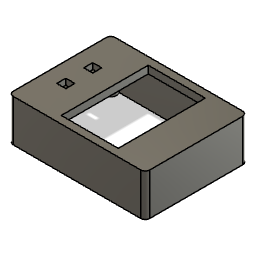
Enclosure_V2 (Autodesk Fusion 360 design; units mm, degrees)
Autodesk Fusion 360 part; units mm, degrees
sketch "Sketch1" plane through (0, 0, 0) normal (0, 1, 0) x (1, 0, 0) in component "Base"
  line L0 (88, -34) -> (-88, -34)
  line L1 (-88, -34) -> (-88, 34)
  line L2 (-88, 34) -> (88, 34)
  line L3 (88, 34) -> (88, -34)
  line L4 (88, -34) -> (-88, 34) construction
  line L5 (-88, -34) -> (88, 34) construction
  line L6 (85.5, -31.5) -> (-85.5, -31.5)
  line L7 (-85.5, -31.5) -> (-85.5, 31.5)
  line L8 (-85.5, 31.5) -> (85.5, 31.5)
  line L9 (85.5, 31.5) -> (85.5, -31.5)
  dimension "d2" = 176
  dimension "d3" = 68
  dimension "d4" = 2.5
  constraint perpendicular L0 L1
  constraint parallel L0 L2
  constraint parallel L1 L3
  constraint horizontal L0
  constraint coincident L4 origin
  constraint coincident L5 origin
  measures "d2" distance of L1.end L2.end
  measures "d3" distance of L0.end L1.end
extrude "Extrude1" add sketch "Sketch1" along normal blind 23 contours L0 L1 L2 L3 | L6 L7 L8 L9 makes body 1 in component "Base"
sketch "Sketch2" plane through (0, 23, 0) normal (0, 1, 0) x (-1, 0, 0) in component "Base"
  line L0 (-88, -34) -> (88, -34)
  line L1 (88, -34) -> (88, 34)
  line L2 (88, 34) -> (-88, 34)
  line L3 (-88, 34) -> (-88, -34)
  line L4 (85.5, 31.5) -> (-85.5, 31.5)
  line L5 (-85.5, 31.5) -> (-85.5, -31.5)
  line L6 (-85.5, -31.5) -> (85.5, -31.5)
  line L7 (85.5, -31.5) -> (85.5, 31.5)
  circle A0 centre (-83, -29) radius 2
  circle A1 centre (-83, 29) radius 2
  circle A2 centre (0, 29) radius 2
  circle A3 centre (0, -29) radius 2
  circle A4 centre (83, -29) radius 2
  circle A5 centre (83, 29) radius 2
  dimension "d7" = -2.5
  dimension "d62" = 4
  dimension "d63" = 5
  dimension "d64" = 5
  dimension "d65" = 4
  dimension "d66" = 5
  dimension "d67" = 5
  dimension "d68" = 4
  dimension "d69" = 5
  dimension "d70" = 4
  dimension "d71" = 5
  dimension "d72" = 4
  dimension "d73" = 5
  dimension "d74" = 5
  dimension "d75" = 4
  dimension "d76" = 5
  dimension "d77" = 5
  measures "d62" diameter of A0
  measures "d63" distance of L0 A0.centre
  measures "d64" distance of L3 A0.centre
  measures "d65" diameter of A1
  measures "d66" distance of L3 A1.centre
  measures "d67" distance of L2 A1.centre
  measures "d68" diameter of A2
  measures "d69" distance of L2 A2.centre
  measures "d70" diameter of A3
  measures "d71" distance of L0 A3.centre
  measures "d72" diameter of A4
  measures "d73" distance of L0 A4.centre
  measures "d74" distance of L1 A4.centre
  measures "d75" diameter of A5
  measures "d76" distance of L2 A5.centre
  measures "d77" distance of L1 A5.centre
extrude "Extrude2" cut sketch "Sketch2" against normal up to surface (19 mm away) contours L4 L5 L6 L7 | A0 | A1 | A2 | A3 | A4 | A5 bodies 1 in component "Base"
fillet "Fillet1" radius 2 4 edges at (85.5, 13.5, -31.5) (85.5, 13.5, 31.5) (-85.5, 13.5, 31.5) (-85.5, 13.5, -31.5) on bodies 1 in component "Base"
fillet "Fillet2" radius 3 4 edges at (-88, 11.5, 34) (-88, 11.5, -34) (88, 11.5, -34) (88, 11.5, 34) on bodies 1 in component "Base"
sketch "Sketch3" plane through (0, 0, 0) normal (0, -1, 0) x (1, 0, 0) in component "Base"
  arc A0 (88, 31) -> (85, 34) centre (85, 31) ccw
  line L0 (85, 34) -> (-85, 34)
  arc A1 (-85, 34) -> (-88, 31) centre (-85, 31) ccw
  line L1 (-88, 31) -> (-88, -31) construction
  arc A2 (-88, -31) -> (-85, -34) centre (-85, -31) ccw
  line L2 (-85, -34) -> (85, -34)
  arc A3 (85, -34) -> (88, -31) centre (85, -31) ccw
  line L3 (88, -31) -> (88, 31)
sketch "Sketch4" plane through (0, 0, 0) normal (0, -1, 0) x (1, 0, 0) in component "Base"
  arc A0 (88, 31) -> (85, 34) centre (85, 31) ccw
  line L0 (85, 34) -> (-85, 34)
  arc A1 (-85, 34) -> (-88, 31) centre (-85, 31) ccw
  line L1 (-88, 31) -> (-88, -31)
  arc A2 (-88, -31) -> (-85, -34) centre (-85, -31) ccw
  line L2 (-85, -34) -> (85, -34)
  arc A3 (85, -34) -> (88, -31) centre (85, -31) ccw
  line L3 (88, -31) -> (88, 31)
  circle A4 centre (-61.5, 24) radius 1.75
  line L4 (85, 34) -> (-85, 34)
  circle A5 centre (-61.5, -24.5) radius 1.75
  line L5 (-85, -34) -> (85, -34)
  circle A6 centre (-28.5, 24) radius 1.75
  circle A7 centre (-28.5, -24.5) radius 1.75
  circle A8 centre (-61.5, 24) radius 3.5
  circle A9 centre (-28.5, 24) radius 3.5
  circle A10 centre (-61.5, -24.5) radius 3.5
  circle A11 centre (-28.5, -24.5) radius 3.5
  circle A12 centre (-83, 29) radius 4
  circle A13 centre (-83, 29) radius 2
  circle A14 centre (-83, 29) radius 4
  circle A15 centre (-83, 29) radius 2.1
  circle A16 centre (-83, -29) radius 2
  line L6 (-88, 31) -> (-88, -31)
  circle A17 centre (-83, -29) radius 4
  circle A18 centre (0, 29) radius 4
  circle A19 centre (0, 29) radius 2
  circle A20 centre (0, -29) radius 4
  circle A21 centre (0, -29) radius 2
  circle A22 centre (83, 29) radius 4
  line L7 (88, -31) -> (88, 31)
  circle A23 centre (83, 29) radius 2
  circle A24 centre (83, -29) radius 4
  circle A25 centre (83, -29) radius 2
  dimension "d14" = 3.5
  dimension "d15" = 26.5
  dimension "d16" = 10
  dimension "d17" = 3.5
  dimension "d18" = 26.5
  dimension "d20" = 3.5
  dimension "d21" = 59.5
  dimension "d22" = 10
  dimension "d23" = 3.5
  dimension "d24" = 59.5
  dimension "d26" = 7
  dimension "d27" = 7
  dimension "d28" = 7
  dimension "d29" = 7
  dimension "d36" = 8
  dimension "d37" = 5
  dimension "d38" = 5
  dimension "d39" = 4
  dimension "d40" = 8
  dimension "d41" = 4.2
  dimension "d42" = 4
  dimension "d43" = 5
  dimension "d44" = 5
  dimension "d45" = 8
  dimension "d46" = 8
  dimension "d47" = 5
  dimension "d48" = 4
  dimension "d49" = 8
  dimension "d50" = 5
  dimension "d51" = 4
  dimension "d52" = 8
  dimension "d53" = 5
  dimension "d54" = 5
  dimension "d55" = 4
  dimension "d56" = 8
  dimension "d57" = 5
  dimension "d58" = 5
  dimension "d59" = 4
  dimension "d154" = 48.5
  dimension "d155" = 48.5
  constraint concentric A4 A8
  constraint concentric A6 A9
  constraint concentric A5 A10
  constraint concentric A7 A11
  constraint concentric A12 A13
  constraint concentric A14 A15
  constraint concentric A16 A17
  constraint concentric A18 A19
  constraint concentric A20 A21
  constraint concentric A22 A23
  constraint concentric A24 A25
  measures "d14" diameter of A4
  measures "d15" distance of L1 A4.centre
  measures "d16" distance of A4.centre L4
  measures "d17" diameter of A5
  measures "d18" distance of L1 A5.centre
  measures "d20" diameter of A6
  measures "d21" distance of L1 A6.centre
  measures "d22" distance of L4 A6.centre
  measures "d23" diameter of A7
  measures "d24" distance of L1 A7.centre
  measures "d26" diameter of A8
  measures "d27" diameter of A9
  measures "d28" diameter of A10
  measures "d29" diameter of A11
  measures "d36" diameter of A12
  measures "d37" distance of L4 A12.centre
  measures "d38" distance of L1 A12.centre
  measures "d39" diameter of A13
  measures "d40" diameter of A14
  measures "d41" diameter of A15
  measures "d42" diameter of A16
  measures "d43" distance of A16.centre L6
  measures "d44" distance of L5 A16.centre
  measures "d45" diameter of A17
  measures "d46" diameter of A18
  measures "d47" distance of L0 A18.centre
  measures "d48" diameter of A19
  measures "d49" diameter of A20
  measures "d50" distance of L5 A20.centre
  measures "d51" diameter of A21
  measures "d52" diameter of A22
  measures "d53" distance of A22.centre L7
  measures "d54" distance of L4 A22.centre
  measures "d55" diameter of A23
  measures "d56" diameter of A24
  measures "d57" distance of L3 A24.centre
  measures "d58" distance of L5 A24.centre
  measures "d59" diameter of A25
  measures "d154" distance of A6.centre A7.centre
  measures "d155" distance of A4.centre A5.centre
extrude "Extrude6" add sketch "Sketch4" against normal blind 23 contours A12 A14 | A13 | A15 | A16 | A17 | A18 | A19 | A20 | A21 | A22 | A23 | A24 | A25 bodies 1 in component "Base"
extrude "Extrude4" cut sketch "Sketch4" against normal up to surface (4 mm away) contours A4 | A5 | A6 | A7 bodies 1 in component "Base"
extrude "Extrude5" cut sketch "Sketch4" against normal blind 2.5 contours A8 | A9 | A10 | A11 bodies 1 in component "Base"
sketch "Sketch5" plane through (0, 0, 0) normal (0, -1, 0) x (1, 0, 0) in component "Base"
  circle A0 centre (-28.5, 24) radius 3.5
  circle A1 centre (-61.5, -24.5) radius 3.5
  circle A2 centre (-61.5, 24) radius 3.5
  circle A3 centre (-28.5, -24.5) radius 3.5
  arc A4 (88, 31) -> (85, 34) centre (85, 31) ccw
  line L0 (85, 34) -> (-85, 34)
  arc A5 (-85, 34) -> (-88, 31) centre (-85, 31) ccw
  line L1 (-88, 31) -> (-88, -31)
  arc A6 (-88, -31) -> (-85, -34) centre (-85, -31) ccw
  line L2 (-85, -34) -> (85, -34)
  arc A7 (85, -34) -> (88, -31) centre (85, -31) ccw
  line L3 (88, -31) -> (88, 31)
  line L4 (-2, 25) -> (2, 25)
  line L5 (2, 25) -> (2, -25)
  line L6 (2, -25) -> (-2, -25)
  line L7 (-2, -25) -> (-2, 25)
  constraint horizontal L4
  constraint vertical L5
  constraint horizontal L6
  constraint vertical L7
sketch "Sketch2 (2)" plane through (0, 23, 0) normal (0, 1, 0) x (-1, 0, 0) in component "Lid1"
  arc A0 (-85, 34) -> (-88, 31) centre (-85, 31) ccw
  line L0 (-88, 31) -> (-88, -31)
  arc A1 (-88, -31) -> (-85, -34) centre (-85, -31) ccw
  line L1 (-85, -34) -> (85, -34)
  arc A2 (85, -34) -> (88, -31) centre (85, -31) ccw
  line L2 (88, -31) -> (88, 31)
  arc A3 (88, 31) -> (85, 34) centre (85, 31) ccw
  line L3 (85, 34) -> (-85, 34)
  arc A4 (-85.5, 25.8775) -> (-79.8775, 31.5) centre (-83, 29) ccw
  line L4 (-79.8775, 31.5) -> (-3.1225, 31.5)
  arc A5 (-3.1225, 31.5) -> (3.1225, 31.5) centre (0, 29) ccw
  line L5 (3.1225, 31.5) -> (79.8775, 31.5)
  arc A6 (79.8775, 31.5) -> (85.5, 25.8775) centre (83, 29) ccw
  line L6 (85.5, 25.8775) -> (85.5, -25.8775)
  arc A7 (85.5, -25.8775) -> (79.8775, -31.5) centre (83, -29) ccw
  line L7 (79.8775, -31.5) -> (3.1225, -31.5)
  arc A8 (3.1225, -31.5) -> (-3.1225, -31.5) centre (0, -29) ccw
  line L8 (-3.1225, -31.5) -> (-79.8775, -31.5)
  arc A9 (-79.8775, -31.5) -> (-85.5, -25.8775) centre (-83, -29) ccw
  line L9 (-85.5, -25.8775) -> (-85.5, 25.8775)
  line L10 (85, -34) -> (-85, -34)
  arc A10 (85, -34) -> (88, -31) centre (85, -31) ccw
  line L11 (88, 31) -> (88, -31)
  arc A11 (88, 31) -> (85, 34) centre (85, 31) ccw
  line L12 (-85, 34) -> (85, 34)
  line L13 (-88, -31) -> (-88, 31)
  arc A12 (-85, 34) -> (-88, 31) centre (-85, 31) ccw
  arc A13 (-88, -31) -> (-85, -34) centre (-85, -31) ccw
  point P0 (85, -34)
  point P1 (88, -31)
  point P2 (88, 31)
  point P3 (85, 34)
  point P4 (-85, 34)
  point P5 (-88, 31)
  point P6 (-88, -31)
  point P7 (-85, -34)
extrude "Extrude2'" add sketch "Sketch2 (2)" along normal blind 6 separate body contours A0 L0 A1 L1 A2 L2 A3 L3 L10 A10 L11 A11 L12 L13 A12 A13 | A4 L4 A5 L5 A6 L6 A7 L7 A8 L8 A9 L9 makes body 2 in component "Lid1"
sketch "Sketch5 (2)" plane through (0, 23, 0) normal (0, 1, 0) x (-1, 0, 0) in component "Lid1"
  arc A0 (-85, 34) -> (-88, 31) centre (-85, 31) ccw
  line L0 (-88, 31) -> (-88, -31)
  arc A1 (-88, -31) -> (-85, -34) centre (-85, -31) ccw
  line L1 (-85, -34) -> (85, -34)
  arc A2 (85, -34) -> (88, -31) centre (85, -31) ccw
  line L2 (88, -31) -> (88, 31)
  arc A3 (88, 31) -> (85, 34) centre (85, 31) ccw
  line L3 (85, 34) -> (-85, 34)
  arc A4 (-85.5, 25.8775) -> (-79.8775, 31.5) centre (-83, 29) ccw
  line L4 (-79.8775, 31.5) -> (-3.1225, 31.5)
  arc A5 (-3.1225, 31.5) -> (3.1225, 31.5) centre (0, 29) ccw
  line L5 (3.1225, 31.5) -> (79.8775, 31.5)
  arc A6 (79.8775, 31.5) -> (85.5, 25.8775) centre (83, 29) ccw
  line L6 (85.5, 25.8775) -> (85.5, -25.8775)
  arc A7 (85.5, -25.8775) -> (79.8775, -31.5) centre (83, -29) ccw
  line L7 (79.8775, -31.5) -> (3.1225, -31.5)
  arc A8 (3.1225, -31.5) -> (-3.1225, -31.5) centre (0, -29) ccw
  line L8 (-3.1225, -31.5) -> (-79.8775, -31.5)
  arc A9 (-79.8775, -31.5) -> (-85.5, -25.8775) centre (-83, -29) ccw
  line L9 (-85.5, -25.8775) -> (-85.5, 25.8775)
  arc A10 (85.5, -25.8775) -> (79.8775, -31.5) centre (83, -29) ccw
  line L10 (79.8775, -31.5) -> (3.1225, -31.5)
  arc A11 (3.1225, -31.5) -> (-3.1225, -31.5) centre (0, -29) ccw
  line L11 (-3.1225, -31.5) -> (-79.8775, -31.5)
  arc A12 (-79.8775, -31.5) -> (-85.5, -25.8775) centre (-83, -29) ccw
  line L12 (-85.5, -25.8775) -> (-85.5, 25.8775)
  arc A13 (-85.5, 25.8775) -> (-79.8775, 31.5) centre (-83, 29) ccw
  line L13 (-79.8775, 31.5) -> (-3.1225, 31.5)
  arc A14 (-3.1225, 31.5) -> (3.1225, 31.5) centre (0, 29) ccw
  line L14 (3.1225, 31.5) -> (79.8775, 31.5)
  arc A15 (79.8775, 31.5) -> (85.5, 25.8775) centre (83, 29) ccw
  line L15 (85.5, 25.8775) -> (85.5, -25.8775)
  point P0 (79.8775, -31.5)
  point P1 (3.1225, -31.5)
  point P2 (-3.1225, -31.5)
  point P3 (-79.8775, -31.5)
  point P4 (-85.5, -25.8775)
  point P5 (-85.5, 25.8775)
  point P6 (-79.8775, 31.5)
  point P7 (-3.1225, 31.5)
  point P8 (3.1225, 31.5)
  point P9 (79.8775, 31.5)
  point P10 (85.5, -25.8775)
  point P11 (85.5, 25.8775)
sketch "Sketch6" plane through (0, 23, 0) normal (0, 1, 0) x (-1, 0, 0) in component "Lid1"
  arc A0 (-85, 34) -> (-88, 31) centre (-85, 31) ccw
  line L0 (-88, 31) -> (-88, -31)
  arc A1 (-88, -31) -> (-85, -34) centre (-85, -31) ccw
  line L1 (-85, -34) -> (85, -34)
  arc A2 (85, -34) -> (88, -31) centre (85, -31) ccw
  line L2 (88, -31) -> (88, 31)
  arc A3 (88, 31) -> (85, 34) centre (85, 31) ccw
  line L3 (85, 34) -> (-85, 34)
  arc A4 (-85.5, 25.8775) -> (-79.8775, 31.5) centre (-83, 29) ccw
  line L4 (-79.8775, 31.5) -> (-3.1225, 31.5)
  arc A5 (-3.1225, 31.5) -> (3.1225, 31.5) centre (0, 29) ccw
  line L5 (3.1225, 31.5) -> (79.8775, 31.5)
  arc A6 (79.8775, 31.5) -> (85.5, 25.8775) centre (83, 29) ccw
  line L6 (85.5, 25.8775) -> (85.5, -25.8775)
  arc A7 (85.5, -25.8775) -> (79.8775, -31.5) centre (83, -29) ccw
  line L7 (79.8775, -31.5) -> (3.1225, -31.5)
  arc A8 (3.1225, -31.5) -> (-3.1225, -31.5) centre (0, -29) ccw
  line L8 (-3.1225, -31.5) -> (-79.8775, -31.5)
  arc A9 (-79.8775, -31.5) -> (-85.5, -25.8775) centre (-83, -29) ccw
  line L9 (-85.5, -25.8775) -> (-85.5, 25.8775)
  line L10 (0, 25) -> (0, -25)
  constraint midpoint A5 L10.start
  constraint midpoint A8 L10.end
extrude "Extrude5'" cut sketch "Sketch6" along normal up to surface (6 mm away) contours A5 L5 A6 L6 A7 L7 A8 L10 bodies 2 in component "Lid1"
extrude "Extrude7" cut sketch "Sketch2" against normal blind 3 contours A0 | A1 | A2 | A3 | A4 | A5 bodies 1 in component "Base"
sketch "Sketch10" plane through (0, 0, 0) normal (0, -1, 0) x (1, 0, 0) in component "Base"
  circle A0 centre (-28.5, 24) radius 3.5
  circle A1 centre (-61.5, -24.5) radius 3.5
  circle A2 centre (-61.5, 24) radius 3.5
  circle A3 centre (-28.5, -24.5) radius 3.5
  arc A4 (88, 31) -> (85, 34) centre (85, 31) ccw
  line L0 (85, 34) -> (-85, 34)
  arc A5 (-85, 34) -> (-88, 31) centre (-85, 31) ccw
  line L1 (-88, 31) -> (-88, -31)
  arc A6 (-88, -31) -> (-85, -34) centre (-85, -31) ccw
  line L2 (-85, -34) -> (85, -34)
  arc A7 (85, -34) -> (88, -31) centre (85, -31) ccw
  line L3 (88, -31) -> (88, 31)
  line L4 (10, 19) -> (25, 19)
  line L5 (25, 19) -> (25, 4)
  line L6 (25, 4) -> (10, 4)
  line L7 (10, 4) -> (10, 19)
  line L8 (88, -31) -> (88, 31)
  line L9 (85, 34) -> (-85, 34)
  dimension "d137" = 15
  dimension "d138" = 15
  dimension "d140" = 78
  dimension "d143" = 15
  constraint horizontal L4
  constraint vertical L5
  constraint horizontal L6
  constraint vertical L7
  measures "d137" distance of L4.start L4.end
  measures "d138" distance of L4.start L6.end
  measures "d140" distance of L7 L8
  measures "d143" distance of L4 L9
extrude "Extrude12" cut sketch "Sketch10" against normal up to surface (4 mm away) contours L4 L5 L6 L7 bodies 1 in component "Base"
sketch "Sketch7" plane through (0, 23, 0) normal (0, 1, 0) x (-1, 0, 0) in component "Lid1"
  circle A0 centre (0, 29) radius 2
  circle A1 centre (83, -29) radius 2
  circle A2 centre (-83, -29) radius 2
  circle A3 centre (0, -29) radius 2
  circle A4 centre (83, 29) radius 2
  circle A5 centre (-83, 29) radius 2
  arc A6 (-85, 34) -> (-88, 31) centre (-85, 31) ccw
  line L0 (-88, 31) -> (-88, -31)
  arc A7 (-88, -31) -> (-85, -34) centre (-85, -31) ccw
  line L1 (-85, -34) -> (85, -34)
  arc A8 (85, -34) -> (88, -31) centre (85, -31) ccw
  line L2 (88, -31) -> (88, 31)
  arc A9 (88, 31) -> (85, 34) centre (85, 31) ccw
  line L3 (85, 34) -> (-85, 34)
  arc A10 (-85.5, 25.8775) -> (-79.8775, 31.5) centre (-83, 29) ccw
  line L4 (-79.8775, 31.5) -> (-3.1225, 31.5)
  arc A11 (-3.1225, 31.5) -> (3.1225, 31.5) centre (0, 29) ccw
  line L5 (3.1225, 31.5) -> (79.8775, 31.5)
  arc A12 (79.8775, 31.5) -> (85.5, 25.8775) centre (83, 29) ccw
  line L6 (85.5, 25.8775) -> (85.5, -25.8775)
  arc A13 (85.5, -25.8775) -> (79.8775, -31.5) centre (83, -29) ccw
  line L7 (79.8775, -31.5) -> (3.1225, -31.5)
  arc A14 (3.1225, -31.5) -> (-3.1225, -31.5) centre (0, -29) ccw
  line L8 (-3.1225, -31.5) -> (-79.8775, -31.5)
  arc A15 (-79.8775, -31.5) -> (-85.5, -25.8775) centre (-83, -29) ccw
  line L9 (-85.5, -25.8775) -> (-85.5, 25.8775)
  circle A16 centre (0, 29) radius 2
  circle A17 centre (-83, 29) radius 2
  circle A18 centre (-83, -29) radius 2
  circle A19 centre (0, -29) radius 2
  circle A20 centre (83, -29) radius 2
  circle A21 centre (83, 29) radius 2
  dimension "d92" = 4
  dimension "d93" = 4
  dimension "d94" = 4
  dimension "d95" = 4
  dimension "d96" = 4
  dimension "d97" = 4
  constraint concentric A0 A16
  constraint concentric A5 A17
  constraint concentric A2 A18
  constraint concentric A3 A19
  constraint concentric A1 A20
  constraint concentric A4 A21
  measures "d92" diameter of A16
  measures "d93" diameter of A17
  measures "d94" diameter of A18
  measures "d95" diameter of A19
  measures "d96" diameter of A20
  measures "d97" diameter of A21
extrude "Extrude4'" cut sketch "Sketch7" along normal blind 3 contours A0 A16 | A1 A20 | A2 A18 | A3 A19 | A4 A21 | A5 A17 bodies 2 in component "Lid1"
sketch "Sketch6 (2)" plane through (0, 0, 0) normal (0, -1, 0) x (1, 0, 0) in component "Base"
  circle A0 centre (-28.5, -24.5) radius 3.5
  circle A1 centre (-61.5, 24) radius 3.5
  circle A2 centre (-61.5, -24.5) radius 3.5
  circle A3 centre (-28.5, 24) radius 3.5
  line L0 (-2, 27) -> (2, 27)
  line L1 (2, 27) -> (2, -27)
  line L2 (2, -27) -> (-2, -27)
  line L3 (-2, -27) -> (-2, 27)
  line L4 (10, 4) -> (10, 19)
  line L5 (10, 19) -> (25, 19)
  line L6 (25, 19) -> (25, 4)
  line L7 (25, 4) -> (10, 4)
  arc A4 (88, 31) -> (85, 34) centre (85, 31) ccw
  line L8 (85, 34) -> (-85, 34)
  arc A5 (-85, 34) -> (-88, 31) centre (-85, 31) ccw
  line L9 (-88, 31) -> (-88, -31)
  arc A6 (-88, -31) -> (-85, -34) centre (-85, -31) ccw
  line L10 (-85, -34) -> (85, -34)
  arc A7 (85, -34) -> (88, -31) centre (85, -31) ccw
  line L11 (88, -31) -> (88, 31)
  constraint horizontal L0
  constraint vertical L1
  constraint horizontal L2
  constraint vertical L3
extrude "Extrude9" add sketch "Sketch6 (2)" against normal blind 23 contours L0 L1 L2 L3 bodies 1 in component "Base"
sketch "Sketch7 (2)" plane through (0, 23, 0) normal (0, 1, 0) x (-1, 0, 0) in component "Base"
  arc A0 (2, 25.5359) -> (3.1225, 31.5) centre (0, 29) ccw
  line L0 (3.1225, 31.5) -> (79.8775, 31.5)
  arc A1 (79.8775, 31.5) -> (85.5, 25.8775) centre (83, 29) ccw
  line L1 (85.5, 25.8775) -> (85.5, -25.8775)
  arc A2 (85.5, -25.8775) -> (79.8775, -31.5) centre (83, -29) ccw
  line L2 (79.8775, -31.5) -> (3.1225, -31.5)
  arc A3 (3.1225, -31.5) -> (2, -25.5359) centre (0, -29) ccw
  line L3 (2, -25.5359) -> (2, 25.5359)
  line L4 (-2, 25.5359) -> (-2, -25.5359)
  arc A4 (-2, -25.5359) -> (-3.1225, -31.5) centre (0, -29) ccw
  line L5 (-3.1225, -31.5) -> (-79.8775, -31.5)
  arc A5 (-79.8775, -31.5) -> (-85.5, -25.8775) centre (-83, -29) ccw
  line L6 (-85.5, -25.8775) -> (-85.5, 25.8775)
  arc A6 (-85.5, 25.8775) -> (-79.8775, 31.5) centre (-83, 29) ccw
  line L7 (-79.8775, 31.5) -> (-3.1225, 31.5)
  arc A7 (-3.1225, 31.5) -> (-2, 25.5359) centre (0, 29) ccw
  circle A8 centre (0, -29) radius 2
  circle A9 centre (0, 29) radius 2
  circle A10 centre (83, -29) radius 2
  circle A11 centre (-83, -29) radius 2
  circle A12 centre (83, 29) radius 2
  circle A13 centre (-83, 29) radius 2
  arc A14 (-85, 34) -> (-88, 31) centre (-85, 31) ccw
  line L8 (-88, 31) -> (-88, -31)
  arc A15 (-88, -31) -> (-85, -34) centre (-85, -31) ccw
  line L9 (-85, -34) -> (85, -34)
  arc A16 (85, -34) -> (88, -31) centre (85, -31) ccw
  line L10 (88, -31) -> (88, 31)
  arc A17 (88, 31) -> (85, 34) centre (85, 31) ccw
  line L11 (85, 34) -> (-85, 34)
  line L12 (2, -17) -> (-2, -17)
  line L13 (-2, -17) -> (-2, -14)
  line L14 (-2, -14) -> (2, -14)
  line L15 (2, -14) -> (2, -17)
  dimension "d120" = 17
  dimension "d121" = 3
  constraint horizontal L12
  constraint vertical L13
  constraint horizontal L14
  constraint vertical L15
  constraint coincident L4 L13.end
  constraint coincident L3 L12.start
  measures "d120" distance of L9 L12
  measures "d121" distance of L12 L14
extrude "Extrude10" cut sketch "Sketch7 (2)" against normal up to surface (19 mm away) contours L3 L4 L12 L13 L14 L15 bodies 1 in component "Base"
sketch "Sketch8" plane through (0, 0, 0) normal (0, -1, 0) x (1, 0, 0) in component "Base"
  circle A0 centre (-28.5, -24.5) radius 3.5
  circle A1 centre (-61.5, 24) radius 3.5
  circle A2 centre (-61.5, -24.5) radius 3.5
  circle A3 centre (-28.5, 24) radius 3.5
  line L0 (8, 27) -> (78, 27)
  line L1 (78, 27) -> (78, 24)
  line L2 (78, 24) -> (8, 24)
  line L3 (8, 24) -> (8, 27)
  line L4 (8, -27) -> (78, -27)
  line L5 (78, -27) -> (78, -24)
  line L6 (78, -24) -> (8, -24)
  line L7 (8, -24) -> (8, -27)
  line L8 (85, 34) -> (-85, 34)
  line L9 (88, -31) -> (88, 31)
  line L10 (-85, -34) -> (85, -34)
  line L11 (78, 27) -> (81, 27)
  line L12 (81, 27) -> (81, -27)
  line L13 (81, -27) -> (78, -27)
  line L14 (78, -27) -> (78, 27)
  line L15 (10, 4) -> (10, 19)
  line L16 (10, 19) -> (25, 19)
  line L17 (25, 19) -> (25, 4)
  line L18 (25, 4) -> (10, 4)
  arc A4 (88, 31) -> (85, 34) centre (85, 31) ccw
  line L19 (85, 34) -> (-85, 34)
  arc A5 (-85, 34) -> (-88, 31) centre (-85, 31) ccw
  line L20 (-88, 31) -> (-88, -31)
  arc A6 (-88, -31) -> (-85, -34) centre (-85, -31) ccw
  line L21 (-85, -34) -> (85, -34)
  arc A7 (85, -34) -> (88, -31) centre (85, -31) ccw
  line L22 (88, -31) -> (88, 31)
  dimension "d122" = 10
  dimension "d123" = 3
  dimension "d124" = 10
  dimension "d125" = 80
  dimension "d126" = 10
  dimension "d127" = 3
  dimension "d128" = 10
  dimension "d129" = 80
  dimension "d130" = 3
  constraint horizontal L0
  constraint vertical L1
  constraint horizontal L2
  constraint vertical L3
  constraint horizontal L4
  constraint vertical L5
  constraint horizontal L6
  constraint vertical L7
  constraint horizontal L11
  constraint vertical L12
  constraint horizontal L13
  constraint vertical L14
  measures "d122" distance of L2 L8
  measures "d123" distance of L0 L2
  measures "d124" distance of L1 L9
  measures "d125" distance of L3 L9
  measures "d126" distance of L6 L10
  measures "d127" distance of L4 L6
  measures "d128" distance of L5 L9
  measures "d129" distance of L7 L9
  measures "d130" distance of L0.end L11.end
extrude "Extrude11" add sketch "Sketch8" against normal blind 10 contours L0 L1 L2 L3 L14 | L1 L5 L11 L12 L13 L14 | L4 L5 L6 L7 L14 bodies 1 in component "Base"
sketch "Sketch1 (2)" plane through (0, 29, 0) normal (0, 1, 0) x (-1, 0, 0) in component "Lid2"
  line L0 (79.8775, -31.5) -> (3.1225, -31.5)
  arc A0 (3.1225, -31.5) -> (0, -25) centre (0, -29) ccw
  line L1 (0, -25) -> (0, 25)
  arc A1 (0, 25) -> (3.1225, 31.5) centre (0, 29) ccw
  line L2 (3.1225, 31.5) -> (79.8775, 31.5)
  arc A2 (79.8775, 31.5) -> (85.5, 25.8775) centre (83, 29) ccw
  line L3 (85.5, 25.8775) -> (85.5, -25.8775)
  arc A3 (85.5, -25.8775) -> (79.8775, -31.5) centre (83, -29) ccw
  arc A4 (-85, 34) -> (-88, 31) centre (-85, 31) ccw
  line L4 (-88, 31) -> (-88, -31)
  arc A5 (-88, -31) -> (-85, -34) centre (-85, -31) ccw
  line L5 (-85, -34) -> (85, -34)
  arc A6 (85, -34) -> (88, -31) centre (85, -31) ccw
  line L6 (88, -31) -> (88, 31)
  arc A7 (88, 31) -> (85, 34) centre (85, 31) ccw
  line L7 (85, 34) -> (-85, 34)
  line L8 (-85, -34) -> (85, -34)
  arc A8 (-88, -31) -> (-85, -34) centre (-85, -31) ccw
  line L9 (-88, 31) -> (-88, -31)
  arc A9 (-85, 34) -> (-88, 31) centre (-85, 31) ccw
  line L10 (85, 34) -> (-85, 34)
  arc A10 (88, 31) -> (85, 34) centre (85, 31) ccw
  line L11 (88, -31) -> (88, 31)
  arc A11 (85.5, -25.8775) -> (79.8775, -31.5) centre (83, -29) ccw
  line L12 (79.8775, -31.5) -> (3.1225, -31.5)
  arc A12 (85, -34) -> (88, -31) centre (85, -31) ccw
  line L13 (85.5, 25.8775) -> (85.5, -25.8775)
  arc A13 (79.8775, 31.5) -> (85.5, 25.8775) centre (83, 29) ccw
  line L14 (3.1225, 31.5) -> (79.8775, 31.5)
  arc A14 (0, 25) -> (3.1225, 31.5) centre (0, 29) ccw
  line L15 (0, -25) -> (0, 25)
  arc A15 (3.1225, -31.5) -> (0, -25) centre (0, -29) ccw
  line L16 (-3, -34) -> (-3, 34)
  point P0 (85, -34)
  point P1 (-85, -34)
  point P2 (-88, -31)
  point P3 (-88, 31)
  point P4 (-85, 34)
  point P5 (85, 34)
  point P6 (88, 31)
  point P7 (79.8775, -31.5)
  point P8 (88, -31)
  point P9 (85.5, -25.8775)
  point P10 (85.5, 25.8775)
  point P11 (79.8775, 31.5)
  point P12 (3.1225, 31.5)
  point P13 (0, 25)
  point P14 (0, -25)
  point P15 (3.1225, -31.5)
  dimension "d156" = 3
  constraint coincident L8 L16.start
  constraint perpendicular L8 L16
  constraint coincident L10 L16.end
  measures "d156" distance of L15 L16
extrude "Extrude1'" add sketch "Sketch1 (2)" along normal blind 23 separate body contours L5 A6 L6 A7 L7 L8 L10 A10 L11 A12 L16 makes body 3 in component "Lid2"
fillet "Fillet1'" radius 3 2 edges at (3, 40.5, 34) (3, 40.5, -34) on bodies 3 in component "Lid2"
sketch "Sketch2 (3)" plane through (0, 52, 0) normal (0, 1, 0) x (-1, 0, 0) in component "Lid2"
  arc A0 (-3, -31) -> (0, -34) centre (0, -31) ccw
  line L0 (0, -34) -> (85, -34)
  arc A1 (85, -34) -> (88, -31) centre (85, -31) ccw
  line L1 (88, -31) -> (88, 31)
  arc A2 (88, 31) -> (85, 34) centre (85, 31) ccw
  line L2 (85, 34) -> (0, 34)
  arc A3 (0, 34) -> (-3, 31) centre (0, 31) ccw
  line L3 (-3, 31) -> (-3, -31)
  line L4 (79.8775, -31.5) -> (3.1225, -31.5)
  arc A4 (3.1225, -31.5) -> (0, -25) centre (0, -29) ccw
  line L5 (0, -25) -> (0, 25)
  arc A5 (0, 25) -> (3.1225, 31.5) centre (0, 29) ccw
  line L6 (3.1225, 31.5) -> (79.8775, 31.5)
  arc A6 (79.8775, 31.5) -> (85.5, 25.8775) centre (83, 29) ccw
  line L7 (85.5, 25.8775) -> (85.5, -25.8775)
  arc A7 (85.5, -25.8775) -> (79.8775, -31.5) centre (83, -29) ccw
extrude "Extrude2''" add sketch "Sketch2 (3)" along normal blind 5 contours A0 L0 A1 L1 A2 L2 A3 L3 | L4 A4 L5 A5 L6 A6 L7 A7 bodies 3 in component "Lid2"
sketch "Sketch3 (2)" plane through (0, 57, 0) normal (0, 1, 0) x (-1, 0, 0) in component "Lid2"
  line L0 (-3, 31) -> (-3, -31)
  arc A0 (-3, -31) -> (0, -34) centre (0, -31) ccw
  line L1 (0, -34) -> (85, -34)
  arc A1 (85, -34) -> (88, -31) centre (85, -31) ccw
  line L2 (88, -31) -> (88, 31)
  arc A2 (88, 31) -> (85, 34) centre (85, 31) ccw
  line L3 (85, 34) -> (0, 34)
  arc A3 (0, 34) -> (-3, 31) centre (0, 31) ccw
  line L4 (58, -29) -> (20, -29)
  line L5 (20, -29) -> (20, 29)
  line L6 (20, 29) -> (58, 29)
  line L7 (58, 29) -> (58, -29)
  dimension "d162" = 30
  dimension "d163" = 5
  dimension "d164" = 5
  dimension "d165" = 68
  constraint horizontal L4
  constraint vertical L5
  constraint horizontal L6
  constraint vertical L7
  measures "d162" distance of L2 L7
  measures "d163" distance of L3 L6
  measures "d164" distance of L1 L4
  measures "d165" distance of L2 L5
extrude "Extrude3" cut sketch "Sketch3 (2)" against normal up to surface (5 mm away) contours L4 L5 L6 L7 bodies 3 in component "Lid2"
sketch "Sketch5 (3)" plane through (0, 57, 0) normal (0, 1, 0) x (-1, 0, 0) in component "Lid2"
  line L0 (58, 29) -> (58, -29)
  line L1 (58, -29) -> (20, -29)
  line L2 (20, -29) -> (20, 29)
  line L3 (20, 29) -> (58, 29)
  line L4 (-3, 31) -> (-3, -31)
  arc A0 (-3, -31) -> (0, -34) centre (0, -31) ccw
  line L5 (0, -34) -> (85, -34)
  arc A1 (85, -34) -> (88, -31) centre (85, -31) ccw
  line L6 (88, -31) -> (88, 31)
  arc A2 (88, 31) -> (85, 34) centre (85, 31) ccw
  line L7 (85, 34) -> (0, 34)
  arc A3 (0, 34) -> (-3, 31) centre (0, 31) ccw
  line L8 (78, -6) -> (72, -6)
  line L9 (72, -6) -> (72, -12)
  line L10 (72, -12) -> (78, -12)
  line L11 (78, -12) -> (78, -6)
  line L12 (78, 6) -> (72, 6)
  line L13 (72, 6) -> (72, 12)
  line L14 (72, 12) -> (78, 12)
  line L15 (78, 12) -> (78, 6)
  dimension "d176" = 10
  dimension "d177" = 10
  dimension "d178" = 22
  dimension "d179" = 22
  dimension "d189" = 6
  dimension "d190" = 6
  dimension "d191" = 6
  dimension "d192" = 6
  constraint horizontal L8
  constraint vertical L9
  constraint horizontal L10
  constraint vertical L11
  constraint horizontal L12
  constraint vertical L13
  constraint horizontal L14
  constraint vertical L15
  measures "d176" distance of L6 L11
  measures "d177" distance of L6 L15
  measures "d178" distance of L5 L10
  measures "d179" distance of L7 L14
  measures "d189" distance of L9 L11
  measures "d190" distance of L8 L10
  measures "d191" distance of L12 L14
  measures "d192" distance of L13 L15
extrude "Extrude4''" cut sketch "Sketch5 (3)" against normal blind 4 contours L8 L9 L10 L11 | L12 L13 L14 L15 bodies 3 in component "Lid2"
sketch "Sketch7 (3)" plane through (0, 53, 0) normal (0, 1, 0) x (-1, 0, 0) in component "Lid2"
  line L0 (78, -12) -> (78, -6)
  line L1 (78, -6) -> (72, -6)
  line L2 (72, -6) -> (72, -12)
  line L3 (72, -12) -> (78, -12)
  line L4 (72, -8) -> (78, -8)
  line L5 (78, -8) -> (78, -10)
  line L6 (78, -10) -> (72, -10)
  line L7 (72, -10) -> (72, -8)
  line L8 (88, -31) -> (88, 31)
  dimension "d182" = 2
  dimension "d183" = 6
  dimension "d184" = 10
  constraint horizontal L4
  constraint vertical L5
  constraint horizontal L6
  constraint vertical L7
  measures "d182" distance of L4.start L6.end
  measures "d183" distance of L4.start L4.end
  measures "d184" distance of L5 L8
extrude "Extrude5''" cut sketch "Sketch7 (3)" against normal up to surface (1 mm away) contours L0 L2 L4 L5 L6 L7 bodies 3 in component "Lid2"
sketch "Sketch8 (2)" plane through (0, 53, 0) normal (0, 1, 0) x (-1, 0, 0) in component "Lid2"
  line L0 (78, 12) -> (72, 12)
  line L1 (72, 12) -> (72, 6)
  line L2 (72, 6) -> (78, 6)
  line L3 (78, 6) -> (78, 12)
  line L4 (78, 8) -> (72, 8)
  line L5 (72, 8) -> (72, 10)
  line L6 (72, 10) -> (78, 10)
  line L7 (78, 10) -> (78, 8)
  constraint horizontal L4
  constraint vertical L5
  constraint horizontal L6
  constraint vertical L7
  constraint coincident L1 L5.end
  constraint coincident L3 L4.start
extrude "Extrude6'" cut sketch "Sketch8 (2)" against normal up to surface (1 mm away) contours L1 L3 L4 L5 L6 L7 bodies 3 in component "Lid2"
component "Base" placed x (1, 0, 0) y (0, 1, 0) z (0, 0, 1) at (0, 0, 0)
component "Lid1" placed x (1, 0, 0) y (0, 1, 0) z (0, 0, 1) at (0, 0, 0)
component "Lid2" placed x (1, 0, 0) y (0, 1, 0) z (0, 0, 1) at (0, 0, 0)
component "Lid-Lid" placed x (1, 0, 0) y (0, 1, 0) z (0, 0, 1) at (0, 0, 0)
